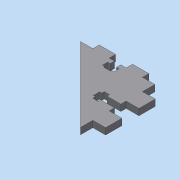
# Autodesk Inventor part: angle
Saved by Autodesk Inventor 2016 SP1 (Build 200210100, 210)
## iProperties
Created: 2016-03-25
Part Number: angle
Material: Generic
Document SubType Name: Modeling
Designer: Mohamed A.
Density: 1 g/cm^3
Appearance: Default
Mass: 1.8375 g
Surface Area: 15.8349 cm^2
Volume: 1.8375 cm^3
Author: Mohamed A.
Autodesk Inventor part; units mm, degrees
ref_plane "YZ Plane" through (0, 0, 0) normal (1, 0, 0) x (0, 1, 0)
ref_plane "XZ Plane" through (0, 0, 0) normal (0, 1, 0) x (-1, 0, 0)
ref_plane "XY Plane" through (0, 0, 0) normal (0, 0, 1) x (1, 0, 0)
sketch "Sketch2" plane through (0, 0, 0) normal (0, 0, 1) x (1, 0, 0)
  line L0 (0, 0) -> (0, -5.8333)
  line L1 (0, -35) -> (-35, 0)
  line L2 (-35, 0) -> (-29.1667, 0)
  line L3 (-5.8333, 0) -> (-5.8333, 3)
  line L4 (-5.8333, 3) -> (-13.5, 3)
  line L5 (-13.5, 3) -> (-13.5, 0)
  line L6 (-21.5, 0) -> (-21.5, 3)
  line L7 (-21.5, 3) -> (-29.1667, 3)
  line L8 (-29.1667, 3) -> (-29.1667, 0)
  line L9 (-17.5, 7.0256) -> (-17.5, -7.5618) construction
  line L10 (-19, 0) -> (-19, -2)
  line L11 (-19, -2) -> (-20.2, -2)
  line L12 (-20.2, -2) -> (-20.2, -4.5)
  line L13 (-20.2, -4.5) -> (-19, -4.5)
  line L14 (-19, -4.5) -> (-19, -5)
  line L15 (-19, -5) -> (-16, -5)
  line L16 (-16, -5) -> (-16, -4.5)
  line L17 (-16, -4.5) -> (-14.8, -4.5)
  line L18 (-14.8, -4.5) -> (-14.8, -2)
  line L19 (-14.8, -2) -> (-16, -2)
  line L20 (-16, 0) -> (-16, -2)
  line L21 (-16, 0) -> (-13.5, 0)
  line L22 (-21.5, 0) -> (-19, 0)
  line L23 (-5.8333, 0) -> (0, 0)
  line L24 (0, -5.8333) -> (6, -5.8333)
  line L25 (6, -5.8333) -> (6, -13.5)
  line L26 (6, -13.5) -> (0, -13.5)
  line L27 (0, -21.5) -> (6, -21.5)
  line L28 (6, -21.5) -> (6, -29.1667)
  line L29 (6, -29.1667) -> (0, -29.1667)
  line L30 (0, -16) -> (-6.5, -16)
  line L31 (-9, -16) -> (-10, -16)
  line L32 (-10, -16) -> (-10, -19)
  line L33 (-10, -19) -> (-9, -19)
  line L34 (-9, -19) -> (-9, -20.2)
  line L35 (-9, -20.2) -> (-6.5, -20.2)
  line L36 (-6.5, -20.2) -> (-6.5, -19)
  line L37 (-6.5, -19) -> (0, -19)
  line L38 (-12.8614, -17.5) -> (7.6104, -17.5) construction
  line L39 (-9, -16) -> (-9, -14.8)
  line L40 (-9, -14.8) -> (-6.5, -14.8)
  line L41 (-6.5, -14.8) -> (-6.5, -16)
  line L42 (0, -13.5) -> (0, -16)
  line L43 (0, -19) -> (0, -21.5)
  line L44 (0, -29.1667) -> (0, -35)
  dimension "d2" = 35
  dimension "d5" = 3
  dimension "d6" = 3
  dimension "d7" = 5
  dimension "d8" = 8
  dimension "d9" = 2.5
  dimension "d10" = 5.4
  dimension "d11" = 8
  dimension "d12" = 23.3333
  dimension "d13" = 35
  dimension "d14" = 6
  dimension "d15" = 3
  dimension "d17" = 16
  dimension "d18" = 2.5
  dimension "d19" = 5.4
  dimension "d20" = 1
  dimension "d21" = 8
  dimension "d22" = 23.3333
  constraints: 90 end point, 59 perpendicular, 25 point on line, 8 vertical, 4 collinear, 2 horizontal, 2 symmetric about line, 1 parallel, 8 other
  measures "d2" distance of L1.end L0.start
  measures "d5" distance between parallel lines of L2 L4
  measures "d6" distance between parallel lines of L20 L10
  measures "d7" distance between parallel lines of L7 L11
  measures "d8" distance between parallel lines of L7 L15
  measures "d9" distance between parallel lines of L13 L11
  measures "d10" distance between parallel lines of L18 L12
  measures "d11" distance between parallel lines of L5 L6
  measures "d12" distance between parallel lines of L3 L8
  measures "d13" distance of L1.start L0.start
  measures "d14" distance between parallel lines of L25 L0
  measures "d15" distance between parallel lines of L37 L30
  measures "d17" distance between parallel lines of L28 L32
  measures "d18" distance between parallel lines of L36 L34
  measures "d19" distance between parallel lines of L35 L40
  measures "d20" distance between parallel lines of L39 L32
  measures "d21" distance between parallel lines of L27 L26
  measures "d22" distance between parallel lines of L29 L24
extrude "Extrusion1" add sketch "Sketch2" along normal blind 3
equation "\"d12\" = 0.666667 * d2"
equation "\"d13\" = d2"
equation "\"d22\" = 0.666667 * d13"
body "Solid1"
